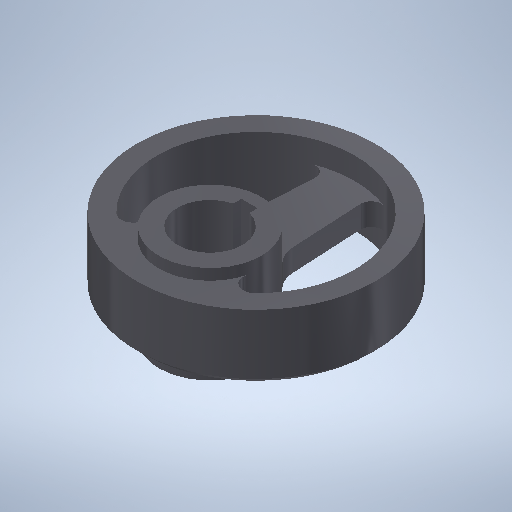
# Autodesk Inventor part: Piesa24_David_Mihai
Saved by Autodesk Inventor 2025 (Build 290162000, 162)
## iProperties
Created: 2023-04-03
Part Number: Piesa24_David_Mihai
Document SubType Name: Modeling
Designer: utilizator
Density: 1 g/cm^3
Material: Generic
Appearance: Steel - Polished
Author: utilizator
Autodesk Inventor part; units mm, degrees
ref_plane "YZ Plane" through (0, 0, 0) normal (1, 0, 0) x (0, 1, 0)
ref_plane "XY Plane" through (0, 0, 0) normal (0, 0, 1) x (1, 0, 0)
sketch "Sketch1" plane through (0, 0, 0) normal (0, 0, 1) x (1, 0, 0)
  circle A0 centre (0, 0) radius 70
  arc A1 (40.7232, -41.2992) -> (-40.7232, -41.2992) centre (0, 0) ccw
  arc A2 (-4.75, -8.6033) -> (4.75, -8.6033) centre (0, -27) ccw
  circle A3 centre (0, -27) radius 30
  arc A4 (29.0338, -34.5526) -> (40.7232, -41.2992) centre (35.8083, -36.3148) ccw
  arc A5 (-40.7232, -41.2992) -> (-29.0338, -34.5526) centre (-35.8083, -36.3148) ccw
  line L0 (0, -46) -> (0, -3.8) construction
  line L1 (-4.75, -3.8) -> (4.75, -3.8)
  line L2 (-4.75, -3.8) -> (-4.75, -8.6033)
  line L3 (4.75, -3.8) -> (4.75, -8.6033)
  line L4 (-19, 54.7996) -> (19, 54.7996) construction
  line L5 (-32.5, 20.2582) -> (32.5, 20.2582) construction
  line L6 (0, -98) -> (0, 98) construction
  arc A6 (15.5233, 6.0625) -> (20.7447, -5.3284) centre (32.5, 6.9522) ccw
  arc A7 (21.5482, 53.8486) -> (13.3273, 47.9641) centre (19.3191, 48.2781) ccw
  line L7 (13.3273, 47.9641) -> (15.5233, 6.0625)
  arc A8 (-13.3273, 47.9641) -> (-21.5482, 53.8486) centre (-19.3191, 48.2781) ccw
  arc A9 (-20.7447, -5.3284) -> (-15.5233, 6.0625) centre (-32.5, 6.9522) ccw
  line L8 (-13.3273, 47.9641) -> (-15.5233, 6.0625)
  point P0 (0, -3.8)
  point P1 (0, 20.2582)
  dimension "d0" = 70
  dimension "d1" = 58
  dimension "d2" = 19
  dimension "d3" = 30
  dimension "d4" = 27
  dimension "d5" = 42.2
  dimension "d6" = 9.5
  dimension "d7" = 38
  dimension "d8" = 65
  dimension "d13" = 7
  dimension "d14" = 7
  dimension "d15" = 3.8
  dimension "d16" = 17
  dimension "d17" = 6
  dimension "d18" = 3
  dimension "d19" = 6
  dimension "d20" = 17
  dimension "d21" = 3
  constraints: 25 point on circle, 16 end point, 12 tangent, 10 centre point, 6 vertical alignment, 3 coincident, 3 perpendicular, 2 midpoint, 2 parallel, 1 vertical
  measures "d0" radius of A0
  measures "d1" radius of A1
  measures "d2" radius of A2
  measures "d3" radius of A3
  measures "d4" distance of A3.centre A1.centre
  measures "d5" distance of L0.start L0.end
  measures "d6" distance of L1.start L1.end
  measures "d7" distance of L4.start L4.end
  measures "d8" distance of L5.start L5.end
  measures "d13" radius of A5
  measures "d14" radius of A4
  measures "d15" distance from line of point (0, 0) L1
  measures "d16" radius of A6
  measures "d17" radius of A7
  measures "d18" angle of L6 L7
  measures "d19" radius of A8
  measures "d20" radius of A9
  measures "d21" angle of L6 L8
extrude "Extrusion1" add sketch "Sketch1" along normal mid plane 57.15 contours A3
ref_plane "Work Plane1" through (0, 3, 0) normal (0, 1, 0) x (-1, 0, 0)
sketch "Sketch2" plane through (0, 3, 0) normal (0, 1, 0) x (-1, 0, 0)
  line L0 (30, -28.575) -> (-30, -28.575) projected
  line L1 (-30, 28.575) -> (30, 28.575) projected
  line L2 (0, 28.575) -> (0, 9.125)
  line L3 (0, -28.575) -> (0, -3.875)
  point P0 (0, 0)
  dimension "d25" = 19.45
  dimension "d26" = 24.7
  dimension "d27" = 3.875
  dimension "d28" = 9.125
  constraints: 4 end point, 2 midpoint, 1 collinear, 1 perpendicular
  measures "d25" distance of L2.start L2.end
  measures "d26" distance of L3.start L3.end
  measures "d27" distance of L3.end point (0, 0)
  measures "d28" distance of L2.end point (0, 0)
extrude "Extrusion2" add sketch "Sketch1" along normal blind 9.125 and the other way blind 3.875 contours A7 L7 A6 A3 A9 L8 A8 A1
sketch "Sketch3" plane through (0, 3, 0) normal (0, 1, 0) x (-1, 0, 0)
  line L0 (20.7447, -3.875) -> (-20.7447, -3.875) projected
  line L1 (-20.7447, -3.875) -> (-20.7447, 9.125) projected
  line L2 (-20.7447, 9.125) -> (20.7447, 9.125) projected
  line L3 (20.7447, -3.875) -> (20.7447, 9.125) projected
  line L4 (30, -28.575) -> (-30, -28.575) projected
  line L5 (-30, 28.575) -> (30, 28.575) projected
  line L6 (0, 28.575) -> (0, 22.125)
  line L7 (0, -28.575) -> (0, -16.075)
  point P0 (0, 0)
  dimension "d33" = 6.45
  dimension "d34" = 12.5
  dimension "d35" = 22.125
  dimension "d36" = 16.075
  constraints: 4 end point, 2 midpoint, 1 collinear, 1 perpendicular
  measures "d33" distance of L6.start L6.end
  measures "d34" distance of L7.start L7.end
  measures "d35" distance of point (0, 0) L6.end
  measures "d36" distance of point (0, 0) L7.end
extrude "Extrusion3" add sketch "Sketch1" along normal blind 22.125 and the other way blind 16.075 contours A0
chamfer "Chamfer1" distance 3 angle 45 1 edges at (-70, 0, -16.075)
body "Solid1"
